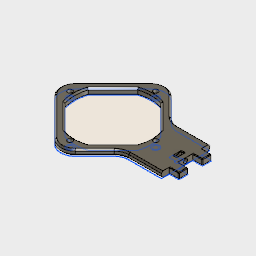
Anet A6 60mm Board Fan holder v2 (Autodesk Fusion 360 design; units mm, degrees)
Autodesk Fusion 360 part; units mm, degrees
note: some values were not read from the file. Set by a fixed rule: which sketch regions a step uses.
sketch "Skizze3" plane through (0, 0, 0) normal (0, 0, 1) x (1, 0, 0)
  line L0 (-4.3, -3) -> (-6.5, -3)
  line L1 (-6.5, -3) -> (-6.5, -1.75)
  line L2 (-6.5, 3) -> (-4.3, 3)
  line L3 (-12, -1.75) -> (-12, 1.75)
  line L4 (-6.5, 1.75) -> (-6.5, 3)
  line L5 (-4.3, -1.75) -> (-4.3, -3)
  line L6 (-4.3, 1.75) -> (0, 1.75)
  line L7 (-6.5, -1.75) -> (-12, -1.75)
  line L8 (0, -1.75) -> (0, -5.85)
  line L9 (-12, 1.75) -> (-6.5, 1.75)
  line L10 (0, -1.75) -> (-4.3, -1.75)
  line L11 (-4.3, 3) -> (-4.3, 1.75)
  line L12 (0, 5.85) -> (0, 1.75)
  line L13 (8, 5.95) -> (0, 5.95)
  line L14 (0, 13.45) -> (8, 13.45)
  line L15 (0, -5.95) -> (8, -5.95)
  line L16 (8, -5.95) -> (8, -13.45)
  line L17 (0, 5.95) -> (0, 1.75)
  line L18 (8, -13.45) -> (0, -13.45)
  line L19 (0, -1.75) -> (0, -5.95)
  line L20 (8, 13.45) -> (8, 5.95)
  line L21 (0, -13.45) -> (8, -13.45)
  line L22 (-90.0032, 9.5948) -> (-69.5948, 30.0032)
  line L23 (-50.4052, 30.0032) -> (-29.9968, 9.5948)
  line L24 (-29.9968, -9.5948) -> (-50.4052, -30.0032)
  line L25 (-69.5948, -30.0032) -> (-90.0032, -9.5948)
  arc A0 (-50.4052, 30.0032) -> (-69.5948, 30.0032) centre (-60, 0) ccw
  arc A1 (-90.0032, 9.5948) -> (-90.0032, -9.5948) centre (-60, 0) ccw
  arc A2 (-69.5948, -30.0032) -> (-50.4052, -30.0032) centre (-60, 0) ccw
  arc A3 (-29.9968, -9.5948) -> (-29.9968, 9.5948) centre (-60, 0) ccw
  line L26 (-99.598, 8.4853) -> (-68.4853, 39.598)
  line L27 (-68.4853, -39.598) -> (-99.598, -8.4853)
  line L28 (-35.4315, -23.5147) -> (-51.5147, -39.598)
  line L29 (-51.5147, 39.598) -> (-35.4315, 23.5147)
  arc A4 (-99.598, 8.4853) -> (-99.598, -8.4853) centre (-91.1127, 0) ccw
  arc A5 (-51.5147, 39.598) -> (-68.4853, 39.598) centre (-60, 31.1127) ccw
  arc A6 (-68.4853, -39.598) -> (-51.5147, -39.598) centre (-60, -31.1127) ccw
  line L30 (0, 13.45) -> (0, 20)
  line L31 (0, 20) -> (-26.9462, 20)
  line L32 (0, -13.45) -> (0, -20)
  line L33 (0, -20) -> (-26.9462, -20)
  arc A7 (-35.4315, 23.5147) -> (-26.9462, 20) centre (-26.9462, 32) ccw
  arc A8 (-26.9462, -20) -> (-35.4315, -23.5147) centre (-26.9462, -32) ccw
  line L34 (-6.5, 1.75) -> (-6.5, -1.75)
  line L35 (-4.3, 1.75) -> (-4.3, -1.75)
  line L36 (0, 1.75) -> (0, -1.75)
  line L37 (0, 13.45) -> (0, 5.95)
  line L38 (0, -5.95) -> (0, -13.45)
  circle A9 centre (-95.3553, 0) radius 3
  circle A10 centre (-60, -35.3553) radius 3
  circle A11 centre (-24.6447, 0) radius 3
  circle A12 centre (-60, 35.3553) radius 3
  circle A13 centre (-60, -35.3553) radius 2
  circle A14 centre (-95.3553, 0) radius 2
  circle A15 centre (-24.6447, 0) radius 2
  circle A16 centre (-60, 35.3553) radius 2
  point P0 (-102.4264, 0)
  point P1 (-60, -42.4264)
  dimension "d10" = 12
  measures "d10" radius of A6
sketch "Skizze8" plane through (0, 0, 0) normal (1, 0, 0) x (0, 1, 0)
  line L0 (20, 0) -> (20, 2)
  line L1 (20, 2) -> (-5.95, 2)
  line L2 (-5.95, 2) -> (-5.95, 0)
  circle A0 centre (0, 2.45) radius 1.65
  line L3 (-5.95, 0) -> (20, 0)
extrude "Extrusion8" add sketch "Skizze3" along normal blind 4.9 contours L0 L1 L2 L3 L4 L5 L6 L7 L8 L9 L10 L11 L12 L17 L19 L26 L27 L28 L29 A4 A5 A6 L30 L31 L32 L33 A7 A8 L37 L38 | L6 L10 L35 L36 | L3 L7 L9 L34 | L15 L16 L18 L21 L38 | L13 L14 L20 L37 | A9 | A10 | A11 | A12
extrude "Extrusion9" cut sketch "Skizze8" against normal blind 13 contours L1 A0 | L1 A0
extrude "Extrusion10" cut sketch "Skizze3" along normal blind 1.8 contours A9 | A10 | A11 | A12
chamfer "Fase3" distance 1.5 angle 45 11 edges at (-13.4731, -20, 0) (-31.5384, -20.9134, 0) (-43.4731, -31.5563, 0) (-60, -43.1127, 0) (-84.0416, -24.0416, 0) (-103.1127, 0, 0) (-84.0416, 24.0416, 0) (-60, 43.1127, 0) (-43.4731, 31.5563, 0) (-31.5384, 20.9134, 0) (-13.4731, 20, 0)
chamfer "Fase4" distance 0.5 angle 45 8 edges at (-60, -31.5, 0) (-79.799, -19.799, 0) (-91.5, 0, 0) (-79.799, 19.799, 0) (-60, 31.5, 0) (-40.201, 19.799, 0) (-28.5, 0, 0) (-40.201, -19.799, 0)
chamfer "Fase5" distance 0.3 angle 45 4 edges at (-62.797, -36.4402, 0) (-27.4416, -1.0848, 0) (-62.797, 34.2705, 0) (-98.1523, -1.0848, 0)
chamfer "Fase6" distance 0.4 angle 45 4 edges at (-5.4, -3, 0) (-6.5, 0, 0) (-5.4, 3, 0) (-4.3, 0, 0)
chamfer "Fase7" distance 0.5 angle 45 6 edges at (4, -13.45, 0) (8, -9.7, 0) (4, -5.95, 0) (4, 5.95, 0) (8, 9.7, 0) (4, 13.45, 0)
chamfer "Fase8" distance 0.5 angle 45 10 edges at (-6.5, 0, 4.9) (-5.4, -3, 4.9) (-4.3, 0, 4.9) (-5.4, 3, 4.9) (4, 13.45, 4.9) (8, 9.7, 4.9) (4, 5.95, 4.9) (4, -5.95, 4.9) (4, -13.45, 4.9) (8, -9.7, 4.9)
chamfer "Fase9" distance 0.5 angle 45 4 edges at (8, 13.45, 2.45) (8, 5.95, 2.45) (8, -5.95, 2.45) (8, -13.45, 2.45)
chamfer "Fase10" distance 1.2 angle 45 8 edges at (-79.799, -19.799, 4.9) (-91.5, 0, 4.9) (-79.799, 19.799, 4.9) (-60, 31.5, 4.9) (-40.201, 19.799, 4.9) (-28.5, 0, 4.9) (-40.201, -19.799, 4.9) (-60, -31.5, 4.9)
chamfer "Fase11" distance 1.2 angle 45 11 edges at (-13.4731, 20, 4.9) (-31.5384, 20.9134, 4.9) (-43.4731, 31.5563, 4.9) (-60, 43.1127, 4.9) (-84.0416, 24.0416, 4.9) (-103.1127, 0, 4.9) (-84.0416, -24.0416, 4.9) (-60, -43.1127, 4.9) (-43.4731, -31.5563, 4.9) (-31.5384, -20.9134, 4.9) (-13.4731, -20, 4.9)
